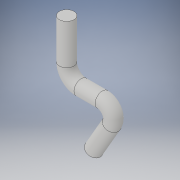
# Autodesk Inventor part: 示範二
Saved by Autodesk Inventor 2017 (Build 210142000, 142)
## iProperties
Part Number: 示範二
Material: 一般
Document SubType Name: Modeling
Designer: user
Density: 1 g/cm^3
Appearance: 預設
Author: user
Autodesk Inventor part; units mm, degrees
ref_plane "YZ Plane" through (0, 0, 0) normal (1, 0, 0) x (0, 1, 0)
ref_plane "XZ Plane" through (0, 0, 0) normal (0, 1, 0) x (-1, 0, 0)
sketch "草圖1" plane through (0, 0, 0) normal (0, 0, 1) x (1, 0, 0)
  line L0 (0, 30) -> (0, 8)
  line L1 (8, 0) -> (19.6077, 0)
  line L2 (24.8038, -9) -> (15, -25.9808)
  arc A0 (0, 8) -> (8, 0) centre (8, 8) ccw
  arc A1 (24.8038, -9) -> (19.6077, 0) centre (19.6077, -6) ccw
  point P0 (0, 0)
  point P1 (30, 0)
  dimension "d0" = 60
  dimension "d1" = 30
  dimension "d2" = 30
  dimension "d3" = 15
  dimension "d4" = 8
  dimension "d5" = 6
  constraints: 6 end point, 4 point on circle, 4 point on line, 4 tangent, 2 centre point, 1 perpendicular, 1 vertical
  measures "d0" angle of L1 L2
  measures "d1" distance from line of point (30, 0) L0
  measures "d2" distance of L0.start point (0, 0)
  measures "d3" horizontal distance of point (30, 0) L2.end
  measures "d4" radius of A0
  measures "d5" radius of A1
ref_plane "工作平面1" through (0, 30, 0) normal (0, -1, 0) x (1, 0, 0)
sketch "草圖2" plane through (0, 30, 0) normal (0, -1, 0) x (1, 0, 0)
  circle A0 centre (0, 0) radius 4
  dimension "d6" = 8
  constraints: 1 centre point, 1 coincident
  measures "d6" diameter of A0
sweep "掃掠1" add profiles "草圖2" path "草圖1"
